Autodesk Inventor part; units mm, degrees
(part 3 of 4)
  line L1892 (-2.7113, 2.6703) -> (-2.8783, 2.4896)
  line L1893 (-2.7113, 2.6703) -> (-2.5443, 2.4896)
  line L1894 (-2.5443, 2.4896) -> (-2.7113, 2.3035)
  line L1895 (-2.8783, 2.4896) -> (-2.7113, 2.3035)
  line L1896 (-3.2281, 2.6703) -> (-3.0611, 2.4896)
  line L1897 (-3.2281, 2.6703) -> (-3.3951, 2.4896)
  line L1898 (-3.0611, 2.4896) -> (-3.2281, 2.3035)
  line L1899 (-3.3951, 2.4896) -> (-3.2281, 2.3035)
  line L1900 (-2.7113, 1.1085) -> (-2.8783, 0.9278)
  line L1901 (-2.7113, 1.1085) -> (-2.5443, 0.9278)
  line L1902 (-2.8783, 0.9278) -> (-2.7113, 0.7417)
  line L1903 (-2.7113, 0.6309) -> (-2.8783, 0.4502)
  line L1904 (-2.7113, 0.6309) -> (-2.5443, 0.4502)
  line L1905 (-2.8783, 0.4502) -> (-2.7113, 0.264)
  line L1906 (-2.5443, 0.4502) -> (-2.7113, 0.264)
  line L1907 (-2.5443, 0.9278) -> (-2.7113, 0.7417)
  line L1908 (-2.7113, 1.7094) -> (-2.8783, 1.5287)
  line L1909 (-2.5443, 1.5287) -> (-2.7113, 1.3425)
  line L1910 (-2.7113, 1.7094) -> (-2.5443, 1.5287)
  line L1911 (-2.8783, 1.5287) -> (-2.7113, 1.3425)
  line L1912 (-4.3118, 1.1085) -> (-4.4788, 0.9278)
  line L1913 (-4.4788, 0.9278) -> (-4.3118, 0.7417)
  line L1914 (-4.3118, 1.1085) -> (-4.1448, 0.9278)
  line L1915 (-4.4788, 0.4502) -> (-4.3118, 0.264)
  line L1916 (-4.1448, 0.4502) -> (-4.3118, 0.264)
  line L1917 (-4.3118, 0.6309) -> (-4.1448, 0.4502)
  line L1918 (-4.1448, 0.9278) -> (-4.3118, 0.7417)
  line L1919 (-4.3118, 0.6309) -> (-4.4788, 0.4502)
  line L1920 (-2.3773, 9.764) -> (-2.5443, 9.5833)
  line L1921 (-2.5443, 9.5833) -> (-2.3773, 9.3971)
  line L1922 (-2.3773, 9.764) -> (-2.2103, 9.5833)
  line L1923 (-2.2103, 9.5833) -> (-2.3773, 9.3971)
  line L1924 (-2.3773, 9.2863) -> (-2.5443, 9.1056)
  line L1925 (-2.5443, 9.1056) -> (-2.3773, 8.9195)
  line L1926 (-2.3773, 9.2863) -> (-2.2103, 9.1056)
  line L1927 (-2.2103, 9.1056) -> (-2.3773, 8.9195)
  line L1928 (-2.3773, 8.827) -> (-2.5443, 8.6463)
  line L1929 (-2.5443, 8.6463) -> (-2.3773, 8.4602)
  line L1930 (-2.3773, 8.827) -> (-2.2103, 8.6463)
  line L1931 (-2.2103, 8.6463) -> (-2.3773, 8.4602)
  line L1932 (-2.3773, 8.3637) -> (-2.5443, 8.183)
  line L1933 (-2.5443, 8.183) -> (-2.3773, 7.9969)
  line L1934 (-2.3773, 8.3637) -> (-2.2103, 8.183)
  line L1935 (-2.2103, 8.183) -> (-2.3773, 7.9969)
  line L1936 (-2.3773, 7.8983) -> (-2.5443, 7.7177)
  line L1937 (-2.5443, 7.7177) -> (-2.3773, 7.5315)
  line L1938 (-2.3773, 7.8983) -> (-2.2103, 7.7177)
  line L1939 (-2.2103, 7.7177) -> (-2.3773, 7.5315)
  line L1940 (-2.3773, 7.4088) -> (-2.5443, 7.2281)
  line L1941 (-2.5443, 7.2281) -> (-2.3773, 7.042)
  line L1942 (-2.3773, 7.4088) -> (-2.2103, 7.2281)
  line L1943 (-2.2103, 7.2281) -> (-2.3773, 7.042)
  line L1944 (-2.3773, 6.9434) -> (-2.5443, 6.7628)
  line L1945 (-2.5443, 6.7628) -> (-2.3773, 6.5766)
  line L1946 (-2.3773, 6.9434) -> (-2.2103, 6.7628)
  line L1947 (-2.2103, 6.7628) -> (-2.3773, 6.5766)
  line L1948 (-2.3773, 6.4539) -> (-2.5443, 6.2732)
  line L1949 (-2.5443, 6.2732) -> (-2.3773, 6.0871)
  line L1950 (-2.3773, 6.4539) -> (-2.2103, 6.2732)
  line L1951 (-2.2103, 6.2732) -> (-2.3773, 6.0871)
  line L1952 (-2.3773, 5.9825) -> (-2.5443, 5.8018)
  line L1953 (-2.5443, 5.8018) -> (-2.3773, 5.6157)
  line L1954 (-2.3773, 5.9825) -> (-2.2103, 5.8018)
  line L1955 (-2.2103, 5.8018) -> (-2.3773, 5.6157)
  line L1956 (-2.3773, 5.4909) -> (-2.5443, 5.3102)
  line L1957 (-2.5443, 5.3102) -> (-2.3773, 5.124)
  line L1958 (-2.3773, 5.4909) -> (-2.2103, 5.3102)
  line L1959 (-2.3773, 4.5539) -> (-2.5443, 4.3732)
  line L1960 (-2.3773, 4.5539) -> (-2.2103, 4.3732)
  line L1961 (-2.5443, 4.8325) -> (-2.3773, 4.6463)
  line L1962 (-2.2103, 4.8325) -> (-2.3773, 4.6463)
  line L1963 (-2.3773, 5.0132) -> (-2.2103, 4.8325)
  line L1964 (-2.2103, 5.3102) -> (-2.3773, 5.124)
  line L1965 (-2.3773, 5.0132) -> (-2.5443, 4.8325)
  line L1966 (-2.5443, 4.3732) -> (-2.3773, 4.187)
  line L1967 (-2.2103, 4.3732) -> (-2.3773, 4.187)
  line L1968 (-2.3773, 4.0906) -> (-2.5443, 3.9099)
  line L1969 (-2.3773, 4.0906) -> (-2.2103, 3.9099)
  line L1970 (-2.5443, 3.9099) -> (-2.3773, 3.7237)
  line L1971 (-2.2103, 3.9099) -> (-2.3773, 3.7237)
  line L1972 (-2.3773, 3.6252) -> (-2.5443, 3.4445)
  line L1973 (-2.3773, 3.6252) -> (-2.2103, 3.4445)
  line L1974 (-2.5443, 3.4445) -> (-2.3773, 3.2584)
  line L1975 (-2.2103, 3.4445) -> (-2.3773, 3.2584)
  line L1976 (-2.3773, 3.1357) -> (-2.5443, 2.955)
  line L1977 (-2.3773, 3.1357) -> (-2.2103, 2.955)
  line L1978 (-2.5443, 2.955) -> (-2.3773, 2.7688)
  line L1979 (-2.2103, 2.955) -> (-2.3773, 2.7688)
  line L1980 (-2.3773, 2.6703) -> (-2.2103, 2.4896)
  line L1981 (-2.3773, 2.6703) -> (-2.5443, 2.4896)
  line L1982 (-2.2103, 2.4896) -> (-2.3773, 2.3035)
  line L1983 (-2.5443, 2.4896) -> (-2.3773, 2.3035)
  line L1984 (-2.3773, 2.1808) -> (-2.5443, 2.0001)
  line L1985 (-2.3773, 2.1808) -> (-2.2103, 2.0001)
  line L1986 (-2.5443, 2.0001) -> (-2.3773, 1.8139)
  line L1987 (-2.2103, 2.0001) -> (-2.3773, 1.8139)
  line L1988 (-2.3773, 1.7094) -> (-2.5443, 1.5287)
  line L1989 (-2.3773, 1.7094) -> (-2.2103, 1.5287)
  line L1990 (-2.5443, 1.5287) -> (-2.3773, 1.3425)
  line L1991 (-2.2103, 1.5287) -> (-2.3773, 1.3425)
  line L1992 (-2.3773, 1.1085) -> (-2.5443, 0.9278)
  line L1993 (-2.5443, 0.9278) -> (-2.3773, 0.7417)
  line L1994 (-2.3773, 1.1085) -> (-2.2103, 0.9278)
  line L1995 (-2.5443, 0.4502) -> (-2.3773, 0.264)
  line L1996 (-2.2103, 0.4502) -> (-2.3773, 0.264)
  line L1997 (-2.3773, 0.6309) -> (-2.2103, 0.4502)
  line L1998 (-2.2103, 0.9278) -> (-2.3773, 0.7417)
  line L1999 (-2.3773, 0.6309) -> (-2.5443, 0.4502)
  line L2000 (-1.8605, 9.764) -> (-2.0275, 9.5833)
  line L2001 (-2.0275, 9.5833) -> (-1.8605, 9.3971)
  line L2002 (-1.8605, 9.764) -> (-1.6935, 9.5833)
  line L2003 (-1.8605, 8.827) -> (-2.0275, 8.6463)
  line L2004 (-1.8605, 8.827) -> (-1.6935, 8.6463)
  line L2005 (-1.6935, 9.1056) -> (-1.8605, 8.9195)
  line L2006 (-1.8605, 9.2863) -> (-2.0275, 9.1056)
  line L2007 (-1.8605, 9.2863) -> (-1.6935, 9.1056)
  line L2008 (-1.6935, 9.5833) -> (-1.8605, 9.3971)
  line L2009 (-2.0275, 9.1056) -> (-1.8605, 8.9195)
  line L2010 (-2.0275, 8.6463) -> (-1.8605, 8.4602)
  line L2011 (-1.6935, 8.6463) -> (-1.8605, 8.4602)
  line L2012 (-1.8605, 8.3637) -> (-2.0275, 8.183)
  line L2013 (-1.8605, 8.3637) -> (-1.6935, 8.183)
  line L2014 (-2.0275, 8.183) -> (-1.8605, 7.9969)
  line L2015 (-1.6935, 8.183) -> (-1.8605, 7.9969)
  line L2016 (-1.8605, 7.8983) -> (-2.0275, 7.7177)
  line L2017 (-2.0275, 7.7177) -> (-1.8605, 7.5315)
  line L2018 (-1.6935, 7.7177) -> (-1.8605, 7.5315)
  line L2019 (-1.8605, 7.8983) -> (-1.6935, 7.7177)
  line L2020 (-1.8605, 7.4088) -> (-1.6935, 7.2281)
  line L2021 (-1.8605, 7.4088) -> (-2.0275, 7.2281)
  line L2022 (-2.0275, 7.2281) -> (-1.8605, 7.042)
  line L2023 (-1.6935, 7.2281) -> (-1.8605, 7.042)
  line L2024 (-1.8605, 6.9434) -> (-1.6935, 6.7628)
  line L2025 (-1.6935, 6.7628) -> (-1.8605, 6.5766)
  line L2026 (-2.0275, 6.7628) -> (-1.8605, 6.5766)
  line L2027 (-1.8605, 6.9434) -> (-2.0275, 6.7628)
  line L2028 (-1.8605, 6.4539) -> (-2.0275, 6.2732)
  line L2029 (-1.8605, 6.4539) -> (-1.6935, 6.2732)
  line L2030 (-2.0275, 6.2732) -> (-1.8605, 6.0871)
  line L2031 (-1.6935, 6.2732) -> (-1.8605, 6.0871)
  line L2032 (-1.8605, 5.9825) -> (-2.0275, 5.8018)
  line L2033 (-1.8605, 5.9825) -> (-1.6935, 5.8018)
  line L2034 (-2.0275, 5.8018) -> (-1.8605, 5.6157)
  line L2035 (-1.6935, 5.8018) -> (-1.8605, 5.6157)
  line L2036 (-1.8605, 5.4909) -> (-2.0275, 5.3102)
  line L2037 (-1.8605, 5.4909) -> (-1.6935, 5.3102)
  line L2038 (-2.0275, 5.3102) -> (-1.8605, 5.124)
  line L2039 (-1.6935, 5.3102) -> (-1.8605, 5.124)
  line L2040 (-1.8605, 5.0132) -> (-2.0275, 4.8325)
  line L2041 (-1.8605, 5.0132) -> (-1.6935, 4.8325)
  line L2042 (-2.0275, 4.8325) -> (-1.8605, 4.6463)
  line L2043 (-1.6935, 4.8325) -> (-1.8605, 4.6463)
  line L2044 (-1.8605, 4.5539) -> (-1.6935, 4.3732)
  line L2045 (-1.8605, 4.5539) -> (-2.0275, 4.3732)
  line L2046 (-2.0275, 4.3732) -> (-1.8605, 4.187)
  line L2047 (-1.6935, 4.3732) -> (-1.8605, 4.187)
  line L2048 (-1.8605, 4.0906) -> (-2.0275, 3.9099)
  line L2049 (-1.8605, 4.0906) -> (-1.6935, 3.9099)
  line L2050 (-2.0275, 3.9099) -> (-1.8605, 3.7237)
  line L2051 (-1.6935, 3.9099) -> (-1.8605, 3.7237)
  line L2052 (-1.8605, 3.6252) -> (-2.0275, 3.4445)
  line L2053 (-1.8605, 3.6252) -> (-1.6935, 3.4445)
  line L2054 (-2.0275, 3.4445) -> (-1.8605, 3.2584)
  line L2055 (-1.6935, 3.4445) -> (-1.8605, 3.2584)
  line L2056 (-1.8605, 3.1357) -> (-2.0275, 2.955)
  line L2057 (-1.8605, 3.1357) -> (-1.6935, 2.955)
  line L2058 (-2.0275, 2.955) -> (-1.8605, 2.7688)
  line L2059 (-1.6935, 2.955) -> (-1.8605, 2.7688)
  line L2060 (-1.8605, 2.6703) -> (-1.6935, 2.4896)
  line L2061 (-1.8605, 2.6703) -> (-2.0275, 2.4896)
  line L2062 (-2.0275, 2.4896) -> (-1.8605, 2.3035)
  line L2063 (-1.6935, 2.4896) -> (-1.8605, 2.3035)
  line L2064 (-1.8605, 1.1085) -> (-2.0275, 0.9278)
  line L2065 (-1.8605, 1.1085) -> (-1.6935, 0.9278)
  line L2066 (-2.0275, 0.9278) -> (-1.8605, 0.7417)
  line L2067 (-1.8605, 0.6309) -> (-1.6935, 0.4502)
  line L2068 (-1.8605, 0.6309) -> (-2.0275, 0.4502)
  line L2069 (-2.0275, 0.4502) -> (-1.8605, 0.264)
  line L2070 (-1.6935, 0.4502) -> (-1.8605, 0.264)
  line L2071 (-1.6935, 0.9278) -> (-1.8605, 0.7417)
  line L2072 (-1.8605, 2.1808) -> (-1.6935, 2.0001)
  line L2073 (-1.8605, 2.1808) -> (-2.0275, 2.0001)
  line L2074 (-2.0275, 2.0001) -> (-1.8605, 1.8139)
  line L2075 (-1.6935, 2.0001) -> (-1.8605, 1.8139)
  line L2076 (-1.8605, 1.7094) -> (-1.6935, 1.5287)
  line L2077 (-1.8605, 1.7094) -> (-2.0275, 1.5287)
  line L2078 (-1.6935, 1.5287) -> (-1.8605, 1.3425)
  line L2079 (-2.0275, 1.5287) -> (-1.8605, 1.3425)
  line L2080 (-0.7767, 9.2863) -> (-0.9437, 9.1056)
  line L2081 (-0.7767, 9.2863) -> (-0.6097, 9.1056)
  line L2082 (-0.6097, 9.1056) -> (-0.7767, 8.9195)
  line L2083 (-0.9437, 9.1056) -> (-0.7767, 8.9195)
  line L2084 (-0.7767, 8.827) -> (-0.6097, 8.6463)
  line L2085 (-0.7767, 8.827) -> (-0.9437, 8.6463)
  line L2086 (-1.2936, 9.2863) -> (-1.1266, 9.1056)
  line L2087 (-1.2936, 9.2863) -> (-1.4605, 9.1056)
  line L2088 (-1.1266, 9.1056) -> (-1.2936, 8.9195)
  line L2089 (-1.4605, 9.1056) -> (-1.2936, 8.9195)
  line L2090 (-1.2936, 9.764) -> (-1.4605, 9.5833)
  line L2091 (-1.4605, 9.5833) -> (-1.2936, 9.3971)
  line L2092 (-1.1266, 9.5833) -> (-1.2936, 9.3971)
  line L2093 (-1.2936, 9.764) -> (-1.1266, 9.5833)
  line L2094 (-0.9437, 9.5833) -> (-0.7767, 9.3971)
  line L2095 (-0.6097, 9.5833) -> (-0.7767, 9.3971)
  line L2096 (-0.7767, 9.764) -> (-0.9437, 9.5833)
  line L2097 (-0.7767, 9.764) -> (-0.6097, 9.5833)
  line L2098 (-1.2936, 7.4088) -> (-1.4605, 7.2281)
  line L2099 (-1.4605, 7.2281) -> (-1.2936, 7.042)
  line L2100 (-1.2936, 6.4539) -> (-1.1266, 6.2732)
  line L2101 (-1.2936, 6.4539) -> (-1.4605, 6.2732)
  line L2102 (-1.1266, 6.2732) -> (-1.2936, 6.0871)
  line L2103 (-1.4605, 6.2732) -> (-1.2936, 6.0871)
  line L2104 (-0.7767, 5.9825) -> (-0.6097, 5.8018)
  line L2105 (-0.7767, 5.9825) -> (-0.9437, 5.8018)
  line L2106 (-0.6097, 5.8018) -> (-0.7767, 5.6157)
  line L2107 (-0.9437, 5.8018) -> (-0.7767, 5.6157)
  line L2108 (-1.2936, 5.9825) -> (-1.1266, 5.8018)
  line L2109 (-1.2936, 5.9825) -> (-1.4605, 5.8018)
  line L2110 (-1.1266, 5.8018) -> (-1.2936, 5.6157)
  line L2111 (-1.4605, 5.8018) -> (-1.2936, 5.6157)
  line L2112 (-0.9437, 4.8325) -> (-0.7767, 4.6463)
  line L2113 (-0.6097, 4.8325) -> (-0.7767, 4.6463)
  line L2114 (-1.2936, 5.0132) -> (-1.1266, 4.8325)
  line L2115 (-1.2936, 5.0132) -> (-1.4605, 4.8325)
  line L2116 (-0.7767, 4.5539) -> (-0.6097, 4.3732)
  line L2117 (-0.7767, 4.5539) -> (-0.9437, 4.3732)
  line L2118 (-1.1266, 4.8325) -> (-1.2936, 4.6463)
  line L2119 (-1.4605, 4.8325) -> (-1.2936, 4.6463)
  line L2120 (-1.2936, 4.5539) -> (-1.1266, 4.3732)
  line L2121 (-1.2936, 4.5539) -> (-1.4605, 4.3732)
  line L2122 (-1.1266, 3.4445) -> (-1.2936, 3.2584)
  line L2123 (-1.4605, 3.4445) -> (-1.2936, 3.2584)
  line L2124 (-1.2936, 3.6252) -> (-1.1266, 3.4445)
  line L2125 (-1.2936, 3.6252) -> (-1.4605, 3.4445)
  line L2126 (-1.4605, 3.9099) -> (-1.2936, 3.7237)
  line L2127 (-1.2936, 4.0906) -> (-1.1266, 3.9099)
  line L2128 (-1.2936, 4.0906) -> (-1.4605, 3.9099)
  line L2129 (-1.1266, 3.9099) -> (-1.2936, 3.7237)
  line L2130 (-1.2936, 8.827) -> (-1.4605, 8.6463)
  line L2131 (-1.4605, 8.6463) -> (-1.2936, 8.4602)
  line L2132 (-1.2936, 8.827) -> (-1.1266, 8.6463)
  line L2133 (-1.1266, 8.6463) -> (-1.2936, 8.4602)
  line L2134 (-1.2936, 8.3637) -> (-1.4605, 8.183)
  line L2135 (-1.4605, 8.183) -> (-1.2936, 7.9969)
  line L2136 (-1.2936, 8.3637) -> (-1.1266, 8.183)
  line L2137 (-0.6097, 8.6463) -> (-0.7767, 8.4602)
  line L2138 (-0.9437, 8.6463) -> (-0.7767, 8.4602)
  line L2139 (-0.7767, 8.3637) -> (-0.6097, 8.183)
  line L2140 (-0.6097, 8.183) -> (-0.7767, 7.9969)
  line L2141 (-0.9437, 8.183) -> (-0.7767, 7.9969)
  line L2142 (-1.1266, 8.183) -> (-1.2936, 7.9969)
  line L2143 (-0.7767, 8.3637) -> (-0.9437, 8.183)
  line L2144 (-1.2936, 7.8983) -> (-1.4605, 7.7177)
  line L2145 (-1.4605, 7.7177) -> (-1.2936, 7.5315)
  line L2146 (-1.2936, 7.4088) -> (-1.1266, 7.2281)
  line L2147 (-1.1266, 7.2281) -> (-1.2936, 7.042)
  line L2148 (-1.1266, 7.7177) -> (-1.2936, 7.5315)
  line L2149 (-1.2936, 7.8983) -> (-1.1266, 7.7177)
  line L2150 (-0.7767, 6.9434) -> (-0.9437, 6.7628)
  line L2151 (-0.7767, 6.9434) -> (-0.6097, 6.7628)
  line L2152 (-0.7767, 7.4088) -> (-0.9437, 7.2281)
  line L2153 (-0.6097, 7.2281) -> (-0.7767, 7.042)
  line L2154 (-0.9437, 7.7177) -> (-0.7767, 7.5315)
  line L2155 (-0.7767, 7.8983) -> (-0.9437, 7.7177)
  line L2156 (-0.7767, 7.8983) -> (-0.6097, 7.7177)
  line L2157 (-0.6097, 7.7177) -> (-0.7767, 7.5315)
  line L2158 (-0.7767, 7.4088) -> (-0.6097, 7.2281)
  line L2159 (-0.9437, 7.2281) -> (-0.7767, 7.042)
  line L2160 (-1.2936, 6.9434) -> (-1.4605, 6.7628)
  line L2161 (-1.4605, 6.7628) -> (-1.2936, 6.5766)
  line L2162 (-1.2936, 6.9434) -> (-1.1266, 6.7628)
  line L2163 (-1.1266, 6.7628) -> (-1.2936, 6.5766)
  line L2164 (-0.9437, 6.2732) -> (-0.7767, 6.0871)
  line L2165 (-0.6097, 6.2732) -> (-0.7767, 6.0871)
  line L2166 (-0.7767, 6.4539) -> (-0.9437, 6.2732)
  line L2167 (-0.7767, 6.4539) -> (-0.6097, 6.2732)
  line L2168 (-0.9437, 6.7628) -> (-0.7767, 6.5766)
  line L2169 (-0.6097, 6.7628) -> (-0.7767, 6.5766)
  line L2170 (-1.2936, 5.4909) -> (-1.4605, 5.3102)
  line L2171 (-1.4605, 5.3102) -> (-1.2936, 5.124)
  line L2172 (-1.2936, 5.4909) -> (-1.1266, 5.3102)
  line L2173 (-0.7767, 5.0132) -> (-0.9437, 4.8325)
  line L2174 (-1.1266, 5.3102) -> (-1.2936, 5.124)
  line L2175 (-0.9437, 5.3102) -> (-0.7767, 5.124)
  line L2176 (-0.6097, 5.3102) -> (-0.7767, 5.124)
  line L2177 (-0.7767, 5.4909) -> (-0.9437, 5.3102)
  line L2178 (-0.7767, 5.4909) -> (-0.6097, 5.3102)
  line L2179 (-0.7767, 5.0132) -> (-0.6097, 4.8325)
  line L2180 (-1.4605, 4.3732) -> (-1.2936, 4.187)
  line L2181 (-1.1266, 4.3732) -> (-1.2936, 4.187)
  line L2182 (-0.9437, 4.3732) -> (-0.7767, 4.187)
  line L2183 (-0.6097, 4.3732) -> (-0.7767, 4.187)
  line L2184 (-0.7767, 4.0906) -> (-0.9437, 3.9099)
  line L2185 (-0.7767, 4.0906) -> (-0.6097, 3.9099)
  line L2186 (-0.6097, 3.9099) -> (-0.7767, 3.7237)
  line L2187 (-0.7767, 3.6252) -> (-0.9437, 3.4445)
  line L2188 (-0.7767, 3.6252) -> (-0.6097, 3.4445)
  line L2189 (-0.9437, 3.4445) -> (-0.7767, 3.2584)
  line L2190 (-0.6097, 3.4445) -> (-0.7767, 3.2584)
  line L2191 (-0.9437, 3.9099) -> (-0.7767, 3.7237)
  line L2192 (-1.2936, 3.1357) -> (-1.4605, 2.955)
  line L2193 (-1.2936, 3.1357) -> (-1.1266, 2.955)
  line L2194 (-1.4605, 2.955) -> (-1.2936, 2.7688)
  line L2195 (-1.1266, 2.955) -> (-1.2936, 2.7688)
  line L2196 (-1.2936, 2.6703) -> (-1.1266, 2.4896)
  line L2197 (-1.2936, 2.6703) -> (-1.4605, 2.4896)
  line L2198 (-1.1266, 2.4896) -> (-1.2936, 2.3035)
  line L2199 (-1.4605, 2.4896) -> (-1.2936, 2.3035)
  line L2200 (-0.7767, 3.1357) -> (-0.9437, 2.955)
  line L2201 (-0.7767, 3.1357) -> (-0.6097, 2.955)
  line L2202 (-0.9437, 2.955) -> (-0.7767, 2.7688)
  line L2203 (-0.6097, 2.955) -> (-0.7767, 2.7688)
  line L2204 (-0.7767, 2.6703) -> (-0.6097, 2.4896)
  line L2205 (-0.7767, 2.6703) -> (-0.9437, 2.4896)
  line L2206 (-0.6097, 2.4896) -> (-0.7767, 2.3035)
  line L2207 (-0.9437, 2.4896) -> (-0.7767, 2.3035)
  line L2208 (-1.2936, 2.1808) -> (-1.4605, 2.0001)
  line L2209 (-1.2936, 2.1808) -> (-1.1266, 2.0001)
  line L2210 (-1.4605, 2.0001) -> (-1.2936, 1.8139)
  line L2211 (-1.1266, 2.0001) -> (-1.2936, 1.8139)
  line L2212 (-1.2936, 1.7094) -> (-1.4605, 1.5287)
  line L2213 (-1.2936, 1.7094) -> (-1.1266, 1.5287)
  line L2214 (-1.4605, 1.5287) -> (-1.2936, 1.3425)
  line L2215 (-1.1266, 1.5287) -> (-1.2936, 1.3425)
  line L2216 (-0.7767, 2.1808) -> (-0.6097, 2.0001)
  line L2217 (-0.7767, 2.1808) -> (-0.9437, 2.0001)
  line L2218 (-0.9437, 2.0001) -> (-0.7767, 1.8139)
  line L2219 (-0.6097, 2.0001) -> (-0.7767, 1.8139)
  line L2220 (-0.7767, 1.7094) -> (-0.6097, 1.5287)
  line L2221 (-0.7767, 1.7094) -> (-0.9437, 1.5287)
  line L2222 (-0.6097, 1.5287) -> (-0.7767, 1.3425)
  line L2223 (-0.9437, 1.5287) -> (-0.7767, 1.3425)
  line L2224 (-1.2936, 1.1085) -> (-1.4605, 0.9278)
  line L2225 (-1.4605, 0.9278) -> (-1.2936, 0.7417)
  line L2226 (-1.2936, 1.1085) -> (-1.1266, 0.9278)
  line L2227 (-1.4605, 0.4502) -> (-1.2936, 0.264)
  line L2228 (-1.1266, 0.4502) -> (-1.2936, 0.264)
  line L2229 (-1.2936, 0.6309) -> (-1.1266, 0.4502)
  line L2230 (-1.1266, 0.9278) -> (-1.2936, 0.7417)
  line L2231 (-1.2936, 0.6309) -> (-1.4605, 0.4502)
  line L2232 (-0.7767, 1.1085) -> (-0.9437, 0.9278)
  line L2233 (-0.7767, 1.1085) -> (-0.6097, 0.9278)
  line L2234 (-0.9437, 0.9278) -> (-0.7767, 0.7417)
  line L2235 (-0.6097, 0.9278) -> (-0.7767, 0.7417)
  line L2236 (-0.7767, 0.6309) -> (-0.6097, 0.4502)
  line L2237 (-0.7767, 0.6309) -> (-0.9437, 0.4502)
  line L2238 (-0.9437, 0.4502) -> (-0.7767, 0.264)
  line L2239 (-0.6097, 0.4502) -> (-0.7767, 0.264)
  line L2240 (-0.124, 8.827) -> (-0.291, 8.6463)
  line L2241 (-0.124, 8.827) -> (0.043, 8.6463)
  line L2242 (-0.291, 8.6463) -> (-0.124, 8.4602)
  line L2243 (0.2259, 8.6463) -> (0.3929, 8.4602)
  line L2244 (0.5599, 8.6463) -> (0.3929, 8.4602)
  line L2245 (0.3929, 8.3637) -> (0.5599, 8.183)
  line L2246 (0.3929, 8.3637) -> (0.2259, 8.183)
  line L2247 (0.043, 8.6463) -> (-0.124, 8.4602)
  line L2248 (-0.291, 9.1056) -> (-0.124, 8.9195)
  line L2249 (0.043, 9.1056) -> (-0.124, 8.9195)
  line L2250 (-0.124, 9.2863) -> (-0.291, 9.1056)
  line L2251 (-0.124, 9.2863) -> (0.043, 9.1056)
  line L2252 (-0.291, 9.5833) -> (-0.124, 9.3971)
  line L2253 (-0.124, 9.764) -> (0.043, 9.5833)
  line L2254 (-0.124, 9.764) -> (-0.291, 9.5833)
  line L2255 (0.043, 9.5833) -> (-0.124, 9.3971)
  line L2256 (0.5599, 7.7177) -> (0.3929, 7.5315)
  line L2257 (-0.291, 5.8018) -> (-0.124, 5.6157)
  line L2258 (0.043, 5.8018) -> (-0.124, 5.6157)
  line L2259 (-0.124, 5.4909) -> (-0.291, 5.3102)
  line L2260 (-0.124, 5.4909) -> (0.043, 5.3102)
  line L2261 (0.3929, 5.4909) -> (0.2259, 5.3102)
  line L2262 (0.043, 5.3102) -> (-0.124, 5.124)
  line L2263 (0.3929, 5.4909) -> (0.5599, 5.3102)
  line L2264 (0.2259, 5.3102) -> (0.3929, 5.124)
  line L2265 (0.5599, 5.3102) -> (0.3929, 5.124)
  line L2266 (-0.291, 5.3102) -> (-0.124, 5.124)
  line L2267 (-0.124, 4.5539) -> (-0.291, 4.3732)
  line L2268 (-0.124, 4.5539) -> (0.043, 4.3732)
  line L2269 (-0.291, 4.8325) -> (-0.124, 4.6463)
  line L2270 (-0.124, 5.0132) -> (0.043, 4.8325)
  line L2271 (0.3929, 5.0132) -> (0.2259, 4.8325)
  line L2272 (0.3929, 5.0132) -> (0.5599, 4.8325)
  line L2273 (-0.124, 5.0132) -> (-0.291, 4.8325)
  line L2274 (0.043, 4.8325) -> (-0.124, 4.6463)
  line L2275 (0.5599, 4.8325) -> (0.3929, 4.6463)
  line L2276 (0.2259, 4.8325) -> (0.3929, 4.6463)
  line L2277 (-0.291, 4.3732) -> (-0.124, 4.187)
  line L2278 (0.043, 4.3732) -> (-0.124, 4.187)
  line L2279 (0.3929, 4.5539) -> (0.2259, 4.3732)
  line L2280 (0.3929, 4.5539) -> (0.5599, 4.3732)
  line L2281 (0.2259, 4.3732) -> (0.3929, 4.187)
  line L2282 (0.5599, 4.3732) -> (0.3929, 4.187)
  line L2283 (0.3929, 2.6703) -> (0.5599, 2.4896)
  line L2284 (0.3929, 2.6703) -> (0.2259, 2.4896)
  line L2285 (0.2259, 2.4896) -> (0.3929, 2.3035)
  line L2286 (0.5599, 2.4896) -> (0.3929, 2.3035)
  line L2287 (0.3929, 2.1808) -> (0.2259, 2.0001)
  line L2288 (0.3929, 2.1808) -> (0.5599, 2.0001)
  line L2289 (0.2259, 2.0001) -> (0.3929, 1.8139)
  line L2290 (0.5599, 2.0001) -> (0.3929, 1.8139)
  line L2291 (0.7928, 2.0001) -> (0.9598, 1.8139)
  line L2292 (0.9598, 1.7094) -> (0.7928, 1.5287)
  line L2293 (0.7928, 1.5287) -> (0.9598, 1.3425)
  line L2294 (1.1268, 1.5287) -> (0.9598, 1.3425)
  line L2295 (0.9598, 1.7094) -> (1.1268, 1.5287)
  line L2296 (0.9598, 2.1808) -> (0.7928, 2.0001)
  line L2297 (1.1268, 2.0001) -> (0.9598, 1.8139)
  line L2298 (0.9598, 2.1808) -> (1.1268, 2.0001)
  line L2299 (0.3929, 0.6309) -> (0.2259, 0.4502)
  line L2300 (0.2259, 0.4502) -> (0.3929, 0.264)
  line L2301 (0.2259, 0.9278) -> (0.3929, 0.7417)
  line L2302 (0.3929, 1.1085) -> (0.2259, 0.9278)
  line L2303 (0.3929, 0.6309) -> (0.5599, 0.4502)
  line L2304 (0.5599, 0.9278) -> (0.3929, 0.7417)
  line L2305 (0.3929, 1.1085) -> (0.5599, 0.9278)
  line L2306 (0.9598, 0.6309) -> (0.7928, 0.4502)
  line L2307 (0.7928, 0.4502) -> (0.9598, 0.264)
  line L2308 (0.7928, 0.9278) -> (0.9598, 0.7417)
  line L2309 (0.9598, 1.1085) -> (0.7928, 0.9278)
  line L2310 (0.9598, 1.1085) -> (1.1268, 0.9278)
  line L2311 (1.1268, 0.9278) -> (0.9598, 0.7417)
  line L2312 (0.9598, 0.6309) -> (1.1268, 0.4502)
  line L2313 (1.1268, 0.4502) -> (0.9598, 0.264)
  line L2314 (0.5599, 0.4502) -> (0.3929, 0.264)
  line L2315 (0.5599, 8.183) -> (0.3929, 7.9969)
  line L2316 (0.2259, 8.183) -> (0.3929, 7.9969)
  line L2317 (-0.124, 8.3637) -> (0.043, 8.183)
  line L2318 (-0.124, 8.3637) -> (-0.291, 8.183)
  line L2319 (0.3929, 7.8983) -> (0.5599, 7.7177)
  line L2320 (0.043, 8.183) -> (-0.124, 7.9969)
  line L2321 (-0.291, 8.183) -> (-0.124, 7.9969)
  line L2322 (0.3929, 7.8983) -> (0.2259, 7.7177)
  line L2323 (-0.124, 7.8983) -> (0.043, 7.7177)
  line L2324 (0.2259, 7.7177) -> (0.3929, 7.5315)
  line L2325 (-0.124, 7.8983) -> (-0.291, 7.7177)
  line L2326 (-0.291, 7.7177) -> (-0.124, 7.5315)
  line L2327 (0.043, 7.7177) -> (-0.124, 7.5315)
  line L2328 (1.1268, 6.7628) -> (0.9598, 6.5766)
  line L2329 (0.9598, 6.9434) -> (1.1268, 6.7628)
  line L2330 (0.9598, 6.4539) -> (0.7928, 6.2732)
  line L2331 (0.7928, 6.2732) -> (0.9598, 6.0871)
  line L2332 (0.9598, 6.4539) -> (1.1268, 6.2732)
  line L2333 (1.3096, 6.7628) -> (1.4766, 6.5766)
  line L2334 (1.4766, 6.9434) -> (1.3096, 6.7628)
  line L2335 (1.4766, 6.9434) -> (1.6436, 6.7628)
  line L2336 (1.6436, 6.7628) -> (1.4766, 6.5766)
  line L2337 (1.4766, 6.4539) -> (1.3096, 6.2732)
  line L2338 (1.4766, 6.4539) -> (1.6436, 6.2732)
  line L2339 (1.1268, 6.2732) -> (0.9598, 6.0871)
  line L2340 (-0.124, 7.4088) -> (-0.291, 7.2281)
  line L2341 (-0.291, 7.2281) -> (-0.124, 7.042)
  line L2342 (-0.124, 7.4088) -> (0.043, 7.2281)
  line L2343 (0.043, 7.2281) -> (-0.124, 7.042)
  line L2344 (0.3929, 7.4088) -> (0.5599, 7.2281)
  line L2345 (0.3929, 7.4088) -> (0.2259, 7.2281)
  line L2346 (0.2259, 7.2281) -> (0.3929, 7.042)
  line L2347 (0.5599, 7.2281) -> (0.3929, 7.042)
  line L2348 (0.7928, 6.7628) -> (0.9598, 6.5766)
  line L2349 (0.5599, 6.7628) -> (0.3929, 6.5766)
  line L2350 (0.3929, 6.9434) -> (0.5599, 6.7628)
  line L2351 (0.2259, 6.7628) -> (0.3929, 6.5766)
  line L2352 (0.3929, 6.9434) -> (0.2259, 6.7628)
  line L2353 (0.9598, 6.9434) -> (0.7928, 6.7628)
  line L2354 (1.4766, 5.9825) -> (1.3096, 5.8018)
  line L2355 (1.3096, 5.8018) -> (1.4766, 5.6157)
  line L2356 (1.6436, 5.8018) -> (1.4766, 5.6157)
  line L2357 (1.4766, 5.9825) -> (1.6436, 5.8018)
  line L2358 (-0.124, 6.9434) -> (-0.291, 6.7628)
  line L2359 (-0.291, 6.7628) -> (-0.124, 6.5766)
  line L2360 (-0.124, 6.9434) -> (0.043, 6.7628)
  line L2361 (0.043, 6.7628) -> (-0.124, 6.5766)
  line L2362 (-0.124, 5.9825) -> (-0.291, 5.8018)
  line L2363 (-0.124, 5.9825) -> (0.043, 5.8018)
  line L2364 (0.043, 6.2732) -> (-0.124, 6.0871)
  line L2365 (-0.124, 6.4539) -> (-0.291, 6.2732)
  line L2366 (-0.124, 6.4539) -> (0.043, 6.2732)
  line L2367 (-0.291, 6.2732) -> (-0.124, 6.0871)
  line L2368 (-0.124, 4.0906) -> (-0.291, 3.9099)
  line L2369 (-0.124, 4.0906) -> (0.043, 3.9099)
  line L2370 (-0.291, 3.9099) -> (-0.124, 3.7237)
  line L2371 (0.043, 3.9099) -> (-0.124, 3.7237)
  line L2372 (0.3929, 4.0906) -> (0.2259, 3.9099)
  line L2373 (0.3929, 4.0906) -> (0.5599, 3.9099)
  line L2374 (0.2259, 3.9099) -> (0.3929, 3.7237)
  line L2375 (0.5599, 3.9099) -> (0.3929, 3.7237)
  line L2376 (0.3929, 3.6252) -> (0.2259, 3.4445)
  line L2377 (0.3929, 3.6252) -> (0.5599, 3.4445)
  line L2378 (0.2259, 3.4445) -> (0.3929, 3.2584)
  line L2379 (0.5599, 3.4445) -> (0.3929, 3.2584)
  line L2380 (0.7928, 3.4445) -> (0.9598, 3.2584)
  line L2381 (0.9598, 3.6252) -> (0.7928, 3.4445)
  line L2382 (-0.124, 2.1808) -> (-0.291, 2.0001)
  line L2383 (-0.124, 2.1808) -> (0.043, 2.0001)
  line L2384 (-0.291, 2.0001) -> (-0.124, 1.8139)
  line L2385 (0.3929, 1.7094) -> (0.5599, 1.5287)
  line L2386 (0.5599, 1.5287) -> (0.3929, 1.3425)
  line L2387 (0.3929, 1.7094) -> (0.2259, 1.5287)
  line L2388 (0.2259, 1.5287) -> (0.3929, 1.3425)
  line L2389 (-0.124, 1.7094) -> (0.043, 1.5287)
  line L2390 (0.043, 1.5287) -> (-0.124, 1.3425)
  line L2391 (-0.124, 1.7094) -> (-0.291, 1.5287)
  line L2392 (-0.291, 1.5287) -> (-0.124, 1.3425)
  line L2393 (0.043, 2.0001) -> (-0.124, 1.8139)
  line L2394 (-0.124, 3.6252) -> (-0.291, 3.4445)
  line L2395 (-0.124, 3.6252) -> (0.043, 3.4445)
  line L2396 (-0.291, 3.4445) -> (-0.124, 3.2584)
  line L2397 (0.043, 3.4445) -> (-0.124, 3.2584)
  line L2398 (-0.124, 3.1357) -> (-0.291, 2.955)
  line L2399 (-0.124, 3.1357) -> (0.043, 2.955)
  line L2400 (-0.291, 2.955) -> (-0.124, 2.7688)
  line L2401 (0.043, 2.4896) -> (-0.124, 2.3035)
  line L2402 (-0.291, 2.4896) -> (-0.124, 2.3035)
  line L2403 (-0.124, 2.6703) -> (0.043, 2.4896)
  line L2404 (-0.124, 2.6703) -> (-0.291, 2.4896)
  line L2405 (0.2259, 2.955) -> (0.3929, 2.7688)
  line L2406 (0.5599, 2.955) -> (0.3929, 2.7688)
  line L2407 (0.3929, 3.1357) -> (0.5599, 2.955)
  line L2408 (0.3929, 3.1357) -> (0.2259, 2.955)
  line L2409 (0.043, 2.955) -> (-0.124, 2.7688)
  line L2410 (0.3929, 9.764) -> (0.2259, 9.5833)
  line L2411 (0.2259, 9.5833) -> (0.3929, 9.3971)
  line L2412 (0.3929, 9.764) -> (0.5599, 9.5833)
  line L2413 (0.3929, 8.827) -> (0.2259, 8.6463)
  line L2414 (0.3929, 8.827) -> (0.5599, 8.6463)
  line L2415 (0.5599, 9.1056) -> (0.3929, 8.9195)
  line L2416 (0.3929, 9.2863) -> (0.2259, 9.1056)
  line L2417 (0.3929, 9.2863) -> (0.5599, 9.1056)
  line L2418 (0.5599, 9.5833) -> (0.3929, 9.3971)
  line L2419 (0.2259, 9.1056) -> (0.3929, 8.9195)
  line L2420 (1.1268, 9.1056) -> (0.9598, 8.9195)
  line L2421 (0.7928, 9.1056) -> (0.9598, 8.9195)
  line L2422 (1.4766, 9.2863) -> (1.3096, 9.1056)
  line L2423 (1.4766, 9.2863) -> (1.6436, 9.1056)
  line L2424 (1.6436, 9.1056) -> (1.4766, 8.9195)
  line L2425 (1.3096, 9.1056) -> (1.4766, 8.9195)
  line L2426 (0.9598, 9.2863) -> (1.1268, 9.1056)
  line L2427 (0.9598, 9.2863) -> (0.7928, 9.1056)
  line L2428 (0.9598, 9.764) -> (0.7928, 9.5833)
  line L2429 (0.7928, 9.5833) -> (0.9598, 9.3971)
  line L2430 (1.1268, 9.5833) -> (0.9598, 9.3971)
  line L2431 (0.9598, 9.764) -> (1.1268, 9.5833)
  line L2432 (1.3096, 9.5833) -> (1.4766, 9.3971)
  line L2433 (1.6436, 9.5833) -> (1.4766, 9.3971)
  line L2434 (1.4766, 9.764) -> (1.3096, 9.5833)
  line L2435 (1.4766, 9.764) -> (1.6436, 9.5833)
  line L2436 (1.4766, 5.4909) -> (1.3096, 5.3102)
  line L2437 (1.4766, 5.4909) -> (1.6436, 5.3102)
  line L2438 (1.3096, 5.3102) -> (1.4766, 5.124)
  line L2439 (1.6436, 5.3102) -> (1.4766, 5.124)
  line L2440 (0.9598, 5.0132) -> (1.1268, 4.8325)
  line L2441 (0.9598, 5.0132) -> (0.7928, 4.8325)
  line L2442 (0.7928, 4.8325) -> (0.9598, 4.6463)
  line L2443 (1.1268, 4.8325) -> (0.9598, 4.6463)
  line L2444 (1.4766, 5.0132) -> (1.3096, 4.8325)
  line L2445 (1.4766, 5.0132) -> (1.6436, 4.8325)
  line L2446 (1.3096, 4.8325) -> (1.4766, 4.6463)
  line L2447 (1.6436, 4.8325) -> (1.4766, 4.6463)
  line L2448 (1.4766, 4.5539) -> (1.6436, 4.3732)
  line L2449 (1.4766, 4.5539) -> (1.3096, 4.3732)
  line L2450 (0.9598, 4.5539) -> (1.1268, 4.3732)
  line L2451 (0.9598, 4.5539) -> (0.7928, 4.3732)
  line L2452 (1.6436, 4.3732) -> (1.4766, 4.187)
  line L2453 (0.7928, 4.3732) -> (0.9598, 4.187)
  line L2454 (1.1268, 4.3732) -> (0.9598, 4.187)
  line L2455 (1.3096, 4.3732) -> (1.4766, 4.187)
  line L2456 (1.4766, 4.0906) -> (1.6436, 3.9099)
  line L2457 (1.4766, 4.0906) -> (1.3096, 3.9099)
  line L2458 (0.9598, 4.0906) -> (1.1268, 3.9099)
  line L2459 (0.9598, 4.0906) -> (0.7928, 3.9099)
  line L2460 (0.9598, 8.827) -> (1.1268, 8.6463)
  line L2461 (0.9598, 8.827) -> (0.7928, 8.6463)
  line L2462 (1.1268, 8.6463) -> (0.9598, 8.4602)
  line L2463 (0.7928, 8.6463) -> (0.9598, 8.4602)
  line L2464 (1.4766, 8.827) -> (1.3096, 8.6463)
  line L2465 (1.4766, 8.827) -> (1.6436, 8.6463)
  line L2466 (1.3096, 8.6463) -> (1.4766, 8.4602)
  line L2467 (1.6436, 8.6463) -> (1.4766, 8.4602)
  line L2468 (0.9598, 8.3637) -> (1.1268, 8.183)
  line L2469 (0.9598, 8.3637) -> (0.7928, 8.183)
  line L2470 (0.7928, 8.183) -> (0.9598, 7.9969)
  line L2471 (1.1268, 8.183) -> (0.9598, 7.9969)
  line L2472 (1.4766, 8.3637) -> (1.3096, 8.183)
  line L2473 (1.4766, 8.3637) -> (1.6436, 8.183)
  line L2474 (1.3096, 8.183) -> (1.4766, 7.9969)
  line L2475 (1.6436, 8.183) -> (1.4766, 7.9969)
  line L2476 (0.9598, 7.8983) -> (0.7928, 7.7177)
  line L2477 (0.7928, 7.7177) -> (0.9598, 7.5315)
  line L2478 (0.9598, 7.8983) -> (1.1268, 7.7177)
  line L2479 (1.1268, 7.7177) -> (0.9598, 7.5315)
  line L2480 (1.4766, 7.8983) -> (1.3096, 7.7177)
  line L2481 (1.3096, 7.7177) -> (1.4766, 7.5315)
  line L2482 (1.4766, 7.8983) -> (1.6436, 7.7177)
  line L2483 (1.6436, 7.7177) -> (1.4766, 7.5315)
  line L2484 (0.9598, 7.4088) -> (0.7928, 7.2281)
  line L2485 (0.7928, 7.2281) -> (0.9598, 7.042)
  line L2486 (1.4766, 7.4088) -> (1.3096, 7.2281)
  line L2487 (1.4766, 7.4088) -> (1.6436, 7.2281)
  line L2488 (0.9598, 7.4088) -> (1.1268, 7.2281)
  line L2489 (1.6436, 7.2281) -> (1.4766, 7.042)
  line L2490 (1.3096, 7.2281) -> (1.4766, 7.042)
  line L2491 (1.1268, 7.2281) -> (0.9598, 7.042)
  line L2492 (1.3096, 6.2732) -> (1.4766, 6.0871)
  line L2493 (1.6436, 6.2732) -> (1.4766, 6.0871)
  line L2494 (0.7928, 3.9099) -> (0.9598, 3.7237)
  line L2495 (1.1268, 3.4445) -> (0.9598, 3.2584)
  line L2496 (0.9598, 3.6252) -> (1.1268, 3.4445)
  line L2497 (1.1268, 3.9099) -> (0.9598, 3.7237)
  line L2498 (1.3096, 3.4445) -> (1.4766, 3.2584)
  line L2499 (1.4766, 3.6252) -> (1.3096, 3.4445)
  line L2500 (1.4766, 3.1357) -> (1.3096, 2.955)
  line L2501 (1.3096, 3.9099) -> (1.4766, 3.7237)
  line L2502 (1.6436, 3.9099) -> (1.4766, 3.7237)
  line L2503 (1.4766, 3.6252) -> (1.6436, 3.4445)
  line L2504 (1.4766, 3.1357) -> (1.6436, 2.955)
  line L2505 (1.6436, 3.4445) -> (1.4766, 3.2584)
  line L2506 (0.3929, 6.4539) -> (0.2259, 6.2732)
  line L2507 (0.3929, 6.4539) -> (0.5599, 6.2732)
  line L2508 (0.2259, 6.2732) -> (0.3929, 6.0871)
  line L2509 (0.9598, 5.9825) -> (1.1268, 5.8018)
  line L2510 (1.1268, 5.8018) -> (0.9598, 5.6157)
  line L2511 (0.9598, 5.9825) -> (0.7928, 5.8018)
  line L2512 (0.7928, 5.8018) -> (0.9598, 5.6157)
  line L2513 (0.9598, 5.4909) -> (1.1268, 5.3102)
  line L2514 (1.1268, 5.3102) -> (0.9598, 5.124)
  line L2515 (0.7928, 5.3102) -> (0.9598, 5.124)
  line L2516 (0.9598, 5.4909) -> (0.7928, 5.3102)
  line L2517 (0.5599, 6.2732) -> (0.3929, 6.0871)
  line L2518 (0.3929, 5.9825) -> (0.5599, 5.8018)
  line L2519 (0.5599, 5.8018) -> (0.3929, 5.6157)
  line L2520 (0.3929, 5.9825) -> (0.2259, 5.8018)
  line L2521 (0.2259, 5.8018) -> (0.3929, 5.6157)
  line L2522 (1.4766, 2.1808) -> (1.6436, 2.0001)
  line L2523 (1.6436, 2.0001) -> (1.4766, 1.8139)
  line L2524 (1.3096, 2.0001) -> (1.4766, 1.8139)
  line L2525 (1.4766, 2.1808) -> (1.3096, 2.0001)
  line L2526 (0.9598, 3.1357) -> (1.1268, 2.955)
  line L2527 (0.9598, 3.1357) -> (0.7928, 2.955)
  line L2528 (1.3096, 2.955) -> (1.4766, 2.7688)
  line L2529 (1.6436, 2.955) -> (1.4766, 2.7688)
  line L2530 (1.1268, 2.955) -> (0.9598, 2.7688)
  line L2531 (0.7928, 2.955) -> (0.9598, 2.7688)
  line L2532 (1.4766, 2.6703) -> (1.3096, 2.4896)
  line L2533 (1.4766, 2.6703) -> (1.6436, 2.4896)
  line L2534 (1.6436, 2.4896) -> (1.4766, 2.3035)
  line L2535 (1.3096, 2.4896) -> (1.4766, 2.3035)
  line L2536 (0.9598, 2.6703) -> (1.1268, 2.4896)
  line L2537 (0.9598, 2.6703) -> (0.7928, 2.4896)
  line L2538 (1.1268, 2.4896) -> (0.9598, 2.3035)
  line L2539 (0.7928, 2.4896) -> (0.9598, 2.3035)
  line L2540 (1.4766, 1.1085) -> (1.3096, 0.9278)
  line L2541 (1.4766, 1.1085) -> (1.6436, 0.9278)
  line L2542 (1.3096, 0.9278) -> (1.4766, 0.7417)
  line L2543 (1.4766, 0.6309) -> (1.3096, 0.4502)
  line L2544 (1.4766, 0.6309) -> (1.6436, 0.4502)
  line L2545 (1.3096, 0.4502) -> (1.4766, 0.264)
  line L2546 (1.6436, 0.4502) -> (1.4766, 0.264)
  line L2547 (1.6436, 0.9278) -> (1.4766, 0.7417)
  line L2548 (1.4766, 1.7094) -> (1.3096, 1.5287)
  line L2549 (1.6436, 1.5287) -> (1.4766, 1.3425)
  line L2550 (1.4766, 1.7094) -> (1.6436, 1.5287)
  line L2551 (1.3096, 1.5287) -> (1.4766, 1.3425)
  line L2552 (-0.124, 1.1085) -> (-0.291, 0.9278)
  line L2553 (-0.291, 0.9278) -> (-0.124, 0.7417)
  line L2554 (-0.124, 1.1085) -> (0.043, 0.9278)
  line L2555 (-0.291, 0.4502) -> (-0.124, 0.264)
  line L2556 (0.043, 0.4502) -> (-0.124, 0.264)
  line L2557 (-0.124, 0.6309) -> (0.043, 0.4502)
  line L2558 (0.043, 0.9278) -> (-0.124, 0.7417)
  line L2559 (-0.124, 0.6309) -> (-0.291, 0.4502)
  line L2560 (1.8106, 9.764) -> (1.6436, 9.5833)
  line L2561 (1.6436, 9.5833) -> (1.8106, 9.3971)
  line L2562 (1.8106, 9.764) -> (1.9776, 9.5833)
  line L2563 (1.9776, 9.5833) -> (1.8106, 9.3971)
  line L2564 (1.8106, 9.2863) -> (1.6436, 9.1056)
  line L2565 (1.6436, 9.1056) -> (1.8106, 8.9195)
  line L2566 (1.8106, 9.2863) -> (1.9776, 9.1056)
  line L2567 (1.9776, 9.1056) -> (1.8106, 8.9195)
  line L2568 (1.8106, 8.827) -> (1.6436, 8.6463)
  line L2569 (1.6436, 8.6463) -> (1.8106, 8.4602)
  line L2570 (1.8106, 8.827) -> (1.9776, 8.6463)
  line L2571 (1.9776, 8.6463) -> (1.8106, 8.4602)
  line L2572 (1.8106, 8.3637) -> (1.6436, 8.183)
  line L2573 (1.6436, 8.183) -> (1.8106, 7.9969)
  line L2574 (1.8106, 8.3637) -> (1.9776, 8.183)
  line L2575 (1.9776, 8.183) -> (1.8106, 7.9969)
  line L2576 (1.8106, 7.8983) -> (1.6436, 7.7177)
  line L2577 (1.6436, 7.7177) -> (1.8106, 7.5315)
  line L2578 (1.8106, 7.8983) -> (1.9776, 7.7177)
  line L2579 (1.9776, 7.7177) -> (1.8106, 7.5315)
  line L2580 (1.8106, 7.4088) -> (1.6436, 7.2281)
  line L2581 (1.6436, 7.2281) -> (1.8106, 7.042)
  line L2582 (1.8106, 7.4088) -> (1.9776, 7.2281)
  line L2583 (1.9776, 7.2281) -> (1.8106, 7.042)
  line L2584 (1.8106, 6.9434) -> (1.6436, 6.7628)
  line L2585 (1.6436, 6.7628) -> (1.8106, 6.5766)
  line L2586 (1.8106, 6.9434) -> (1.9776, 6.7628)
  line L2587 (1.9776, 6.7628) -> (1.8106, 6.5766)
  line L2588 (1.8106, 6.4539) -> (1.6436, 6.2732)
  line L2589 (1.6436, 6.2732) -> (1.8106, 6.0871)
  line L2590 (1.8106, 6.4539) -> (1.9776, 6.2732)
  line L2591 (1.9776, 6.2732) -> (1.8106, 6.0871)
  line L2592 (1.8106, 5.9825) -> (1.6436, 5.8018)
  line L2593 (1.6436, 5.8018) -> (1.8106, 5.6157)
  line L2594 (1.8106, 5.9825) -> (1.9776, 5.8018)
  line L2595 (1.9776, 5.8018) -> (1.8106, 5.6157)
  line L2596 (1.8106, 5.4909) -> (1.6436, 5.3102)
  line L2597 (1.6436, 5.3102) -> (1.8106, 5.124)
  line L2598 (1.8106, 5.4909) -> (1.9776, 5.3102)
  line L2599 (1.8106, 4.5539) -> (1.6436, 4.3732)
  line L2600 (1.8106, 4.5539) -> (1.9776, 4.3732)
  line L2601 (1.6436, 4.8325) -> (1.8106, 4.6463)
  line L2602 (1.9776, 4.8325) -> (1.8106, 4.6463)
  line L2603 (1.8106, 5.0132) -> (1.9776, 4.8325)
  line L2604 (1.9776, 5.3102) -> (1.8106, 5.124)
  line L2605 (1.8106, 5.0132) -> (1.6436, 4.8325)
  line L2606 (1.6436, 4.3732) -> (1.8106, 4.187)
  line L2607 (1.9776, 4.3732) -> (1.8106, 4.187)
  line L2608 (1.8106, 4.0906) -> (1.6436, 3.9099)
  line L2609 (1.8106, 4.0906) -> (1.9776, 3.9099)
  line L2610 (1.6436, 3.9099) -> (1.8106, 3.7237)
  line L2611 (1.9776, 3.9099) -> (1.8106, 3.7237)
  line L2612 (1.8106, 3.6252) -> (1.6436, 3.4445)
  line L2613 (1.8106, 3.6252) -> (1.9776, 3.4445)
  line L2614 (1.6436, 3.4445) -> (1.8106, 3.2584)
  line L2615 (1.9776, 3.4445) -> (1.8106, 3.2584)
  line L2616 (1.8106, 3.1357) -> (1.6436, 2.955)
  line L2617 (1.8106, 3.1357) -> (1.9776, 2.955)
  line L2618 (1.6436, 2.955) -> (1.8106, 2.7688)
  line L2619 (1.9776, 2.955) -> (1.8106, 2.7688)
  line L2620 (1.8106, 2.6703) -> (1.9776, 2.4896)
  line L2621 (1.8106, 2.6703) -> (1.6436, 2.4896)
  line L2622 (1.9776, 2.4896) -> (1.8106, 2.3035)
  line L2623 (1.6436, 2.4896) -> (1.8106, 2.3035)
  line L2624 (1.8106, 2.1808) -> (1.6436, 2.0001)
  line L2625 (1.8106, 2.1808) -> (1.9776, 2.0001)
  line L2626 (1.6436, 2.0001) -> (1.8106, 1.8139)
  line L2627 (1.9776, 2.0001) -> (1.8106, 1.8139)
  line L2628 (1.8106, 1.7094) -> (1.6436, 1.5287)
  line L2629 (1.8106, 1.7094) -> (1.9776, 1.5287)
  line L2630 (1.6436, 1.5287) -> (1.8106, 1.3425)
  line L2631 (1.9776, 1.5287) -> (1.8106, 1.3425)
  line L2632 (1.8106, 1.1085) -> (1.6436, 0.9278)
  line L2633 (1.6436, 0.9278) -> (1.8106, 0.7417)
  line L2634 (1.8106, 1.1085) -> (1.9776, 0.9278)
  line L2635 (1.6436, 0.4502) -> (1.8106, 0.264)
  line L2636 (1.9776, 0.4502) -> (1.8106, 0.264)
  line L2637 (1.8106, 0.6309) -> (1.9776, 0.4502)
  line L2638 (1.9776, 0.9278) -> (1.8106, 0.7417)
  line L2639 (1.8106, 0.6309) -> (1.6436, 0.4502)
  line L2640 (2.3274, 9.764) -> (2.1604, 9.5833)
  line L2641 (2.1604, 9.5833) -> (2.3274, 9.3971)
  line L2642 (2.3274, 9.764) -> (2.4944, 9.5833)
  line L2643 (2.3274, 8.827) -> (2.1604, 8.6463)
  line L2644 (2.3274, 8.827) -> (2.4944, 8.6463)
  line L2645 (2.4944, 9.1056) -> (2.3274, 8.9195)
  line L2646 (2.3274, 9.2863) -> (2.1604, 9.1056)
  line L2647 (2.3274, 9.2863) -> (2.4944, 9.1056)
  line L2648 (2.4944, 9.5833) -> (2.3274, 9.3971)
  line L2649 (2.1604, 9.1056) -> (2.3274, 8.9195)
  line L2650 (2.1604, 8.6463) -> (2.3274, 8.4602)
  line L2651 (2.4944, 8.6463) -> (2.3274, 8.4602)
  line L2652 (2.3274, 8.3637) -> (2.1604, 8.183)
  line L2653 (2.3274, 8.3637) -> (2.4944, 8.183)
  line L2654 (2.1604, 8.183) -> (2.3274, 7.9969)
  line L2655 (2.4944, 8.183) -> (2.3274, 7.9969)
  line L2656 (2.3274, 7.8983) -> (2.1604, 7.7177)
  line L2657 (2.1604, 7.7177) -> (2.3274, 7.5315)
  line L2658 (2.4944, 7.7177) -> (2.3274, 7.5315)
  line L2659 (2.3274, 7.8983) -> (2.4944, 7.7177)
  line L2660 (2.3274, 7.4088) -> (2.4944, 7.2281)
  line L2661 (2.3274, 7.4088) -> (2.1604, 7.2281)
  line L2662 (2.1604, 7.2281) -> (2.3274, 7.042)
  line L2663 (2.4944, 7.2281) -> (2.3274, 7.042)
  line L2664 (2.3274, 6.9434) -> (2.4944, 6.7628)
  line L2665 (2.4944, 6.7628) -> (2.3274, 6.5766)
  line L2666 (2.1604, 6.7628) -> (2.3274, 6.5766)
  line L2667 (2.3274, 6.9434) -> (2.1604, 6.7628)
  line L2668 (2.3274, 6.4539) -> (2.1604, 6.2732)
  line L2669 (2.3274, 6.4539) -> (2.4944, 6.2732)
  line L2670 (2.1604, 6.2732) -> (2.3274, 6.0871)
  line L2671 (2.4944, 6.2732) -> (2.3274, 6.0871)
  line L2672 (2.3274, 5.9825) -> (2.1604, 5.8018)
  line L2673 (2.3274, 5.9825) -> (2.4944, 5.8018)
  line L2674 (2.1604, 5.8018) -> (2.3274, 5.6157)
  line L2675 (2.4944, 5.8018) -> (2.3274, 5.6157)
  line L2676 (2.3274, 5.4909) -> (2.1604, 5.3102)
  line L2677 (2.3274, 5.4909) -> (2.4944, 5.3102)
  line L2678 (2.1604, 5.3102) -> (2.3274, 5.124)
  line L2679 (2.4944, 5.3102) -> (2.3274, 5.124)
  line L2680 (2.3274, 5.0132) -> (2.1604, 4.8325)
  line L2681 (2.3274, 5.0132) -> (2.4944, 4.8325)
  line L2682 (2.1604, 4.8325) -> (2.3274, 4.6463)
  line L2683 (2.4944, 4.8325) -> (2.3274, 4.6463)
  line L2684 (2.3274, 4.5539) -> (2.4944, 4.3732)
  line L2685 (2.3274, 4.5539) -> (2.1604, 4.3732)
  line L2686 (2.1604, 4.3732) -> (2.3274, 4.187)
  line L2687 (2.4944, 4.3732) -> (2.3274, 4.187)
  line L2688 (2.3274, 4.0906) -> (2.1604, 3.9099)
  line L2689 (2.3274, 4.0906) -> (2.4944, 3.9099)
  line L2690 (2.1604, 3.9099) -> (2.3274, 3.7237)
  line L2691 (2.4944, 3.9099) -> (2.3274, 3.7237)
  line L2692 (2.3274, 3.6252) -> (2.1604, 3.4445)
  line L2693 (2.3274, 3.6252) -> (2.4944, 3.4445)
  line L2694 (2.1604, 3.4445) -> (2.3274, 3.2584)
  line L2695 (2.4944, 3.4445) -> (2.3274, 3.2584)
  line L2696 (2.3274, 3.1357) -> (2.1604, 2.955)
  line L2697 (2.3274, 3.1357) -> (2.4944, 2.955)
  line L2698 (2.1604, 2.955) -> (2.3274, 2.7688)
  line L2699 (2.4944, 2.955) -> (2.3274, 2.7688)
  line L2700 (2.3274, 2.6703) -> (2.4944, 2.4896)
  line L2701 (2.3274, 2.6703) -> (2.1604, 2.4896)
  line L2702 (2.1604, 2.4896) -> (2.3274, 2.3035)
  line L2703 (2.4944, 2.4896) -> (2.3274, 2.3035)
  line L2704 (2.3274, 1.1085) -> (2.1604, 0.9278)
  line L2705 (2.3274, 1.1085) -> (2.4944, 0.9278)
  line L2706 (2.1604, 0.9278) -> (2.3274, 0.7417)
  line L2707 (2.3274, 0.6309) -> (2.4944, 0.4502)
  line L2708 (2.3274, 0.6309) -> (2.1604, 0.4502)
  line L2709 (2.1604, 0.4502) -> (2.3274, 0.264)
  line L2710 (2.4944, 0.4502) -> (2.3274, 0.264)
  line L2711 (2.4944, 0.9278) -> (2.3274, 0.7417)
  line L2712 (2.3274, 2.1808) -> (2.4944, 2.0001)
  line L2713 (2.3274, 2.1808) -> (2.1604, 2.0001)
  line L2714 (2.1604, 2.0001) -> (2.3274, 1.8139)
  line L2715 (2.4944, 2.0001) -> (2.3274, 1.8139)
  line L2716 (2.3274, 1.7094) -> (2.4944, 1.5287)
  line L2717 (2.3274, 1.7094) -> (2.1604, 1.5287)
  line L2718 (2.4944, 1.5287) -> (2.3274, 1.3425)
  line L2719 (2.1604, 1.5287) -> (2.3274, 1.3425)
  line L2720 (3.4111, 9.2863) -> (3.2441, 9.1056)
  line L2721 (3.4111, 9.2863) -> (3.5781, 9.1056)
  line L2722 (3.5781, 9.1056) -> (3.4111, 8.9195)
  line L2723 (3.2441, 9.1056) -> (3.4111, 8.9195)
  line L2724 (3.4111, 8.827) -> (3.5781, 8.6463)
  line L2725 (3.4111, 8.827) -> (3.2441, 8.6463)
  line L2726 (2.8943, 9.2863) -> (3.0613, 9.1056)
  line L2727 (2.8943, 9.2863) -> (2.7273, 9.1056)
  line L2728 (3.0613, 9.1056) -> (2.8943, 8.9195)
  line L2729 (2.7273, 9.1056) -> (2.8943, 8.9195)
  line L2730 (2.8943, 9.764) -> (2.7273, 9.5833)
  line L2731 (2.7273, 9.5833) -> (2.8943, 9.3971)
  line L2732 (3.0613, 9.5833) -> (2.8943, 9.3971)
  line L2733 (2.8943, 9.764) -> (3.0613, 9.5833)
  line L2734 (3.2441, 9.5833) -> (3.4111, 9.3971)
  line L2735 (3.5781, 9.5833) -> (3.4111, 9.3971)
  line L2736 (3.4111, 9.764) -> (3.2441, 9.5833)
  line L2737 (3.4111, 9.764) -> (3.5781, 9.5833)
  line L2738 (2.8943, 7.4088) -> (2.7273, 7.2281)
  line L2739 (2.7273, 7.2281) -> (2.8943, 7.042)
  line L2740 (2.8943, 6.4539) -> (3.0613, 6.2732)
  line L2741 (2.8943, 6.4539) -> (2.7273, 6.2732)
  line L2742 (3.0613, 6.2732) -> (2.8943, 6.0871)
  line L2743 (2.7273, 6.2732) -> (2.8943, 6.0871)
  line L2744 (3.4111, 5.9825) -> (3.5781, 5.8018)
  line L2745 (3.4111, 5.9825) -> (3.2441, 5.8018)
  line L2746 (3.5781, 5.8018) -> (3.4111, 5.6157)
  line L2747 (3.2441, 5.8018) -> (3.4111, 5.6157)
  line L2748 (2.8943, 5.9825) -> (3.0613, 5.8018)
  line L2749 (2.8943, 5.9825) -> (2.7273, 5.8018)
  line L2750 (3.0613, 5.8018) -> (2.8943, 5.6157)
  line L2751 (2.7273, 5.8018) -> (2.8943, 5.6157)
  line L2752 (3.2441, 4.8325) -> (3.4111, 4.6463)
  line L2753 (3.5781, 4.8325) -> (3.4111, 4.6463)
  line L2754 (2.8943, 5.0132) -> (3.0613, 4.8325)
  line L2755 (2.8943, 5.0132) -> (2.7273, 4.8325)
  line L2756 (3.4111, 4.5539) -> (3.5781, 4.3732)
  line L2757 (3.4111, 4.5539) -> (3.2441, 4.3732)
  line L2758 (3.0613, 4.8325) -> (2.8943, 4.6463)
  line L2759 (2.7273, 4.8325) -> (2.8943, 4.6463)
  line L2760 (2.8943, 4.5539) -> (3.0613, 4.3732)
  line L2761 (2.8943, 4.5539) -> (2.7273, 4.3732)
  line L2762 (3.0613, 3.4445) -> (2.8943, 3.2584)
  line L2763 (2.7273, 3.4445) -> (2.8943, 3.2584)
  line L2764 (2.8943, 3.6252) -> (3.0613, 3.4445)
  line L2765 (2.8943, 3.6252) -> (2.7273, 3.4445)
  line L2766 (2.7273, 3.9099) -> (2.8943, 3.7237)
  line L2767 (2.8943, 4.0906) -> (3.0613, 3.9099)
  line L2768 (2.8943, 4.0906) -> (2.7273, 3.9099)
  line L2769 (3.0613, 3.9099) -> (2.8943, 3.7237)
  line L2770 (2.8943, 8.827) -> (2.7273, 8.6463)
  line L2771 (2.7273, 8.6463) -> (2.8943, 8.4602)
  line L2772 (2.8943, 8.827) -> (3.0613, 8.6463)
  line L2773 (3.0613, 8.6463) -> (2.8943, 8.4602)
  line L2774 (2.8943, 8.3637) -> (2.7273, 8.183)
  line L2775 (2.7273, 8.183) -> (2.8943, 7.9969)
  line L2776 (2.8943, 8.3637) -> (3.0613, 8.183)
  line L2777 (3.5781, 8.6463) -> (3.4111, 8.4602)
  line L2778 (3.2441, 8.6463) -> (3.4111, 8.4602)
  line L2779 (3.4111, 8.3637) -> (3.5781, 8.183)
  line L2780 (3.5781, 8.183) -> (3.4111, 7.9969)
  line L2781 (3.2441, 8.183) -> (3.4111, 7.9969)
  line L2782 (3.0613, 8.183) -> (2.8943, 7.9969)
  line L2783 (3.4111, 8.3637) -> (3.2441, 8.183)
  line L2784 (2.8943, 7.8983) -> (2.7273, 7.7177)
  line L2785 (2.7273, 7.7177) -> (2.8943, 7.5315)
  line L2786 (2.8943, 7.4088) -> (3.0613, 7.2281)
  line L2787 (3.0613, 7.2281) -> (2.8943, 7.042)
  line L2788 (3.0613, 7.7177) -> (2.8943, 7.5315)
  line L2789 (2.8943, 7.8983) -> (3.0613, 7.7177)
  line L2790 (3.4111, 6.9434) -> (3.2441, 6.7628)
  line L2791 (3.4111, 6.9434) -> (3.5781, 6.7628)
  line L2792 (3.4111, 7.4088) -> (3.2441, 7.2281)
  line L2793 (3.5781, 7.2281) -> (3.4111, 7.042)
  line L2794 (3.2441, 7.7177) -> (3.4111, 7.5315)
  line L2795 (3.4111, 7.8983) -> (3.2441, 7.7177)
  line L2796 (3.4111, 7.8983) -> (3.5781, 7.7177)
  line L2797 (3.5781, 7.7177) -> (3.4111, 7.5315)
  line L2798 (3.4111, 7.4088) -> (3.5781, 7.2281)
  line L2799 (3.2441, 7.2281) -> (3.4111, 7.042)
  line L2800 (2.8943, 6.9434) -> (2.7273, 6.7628)
  line L2801 (2.7273, 6.7628) -> (2.8943, 6.5766)
  line L2802 (2.8943, 6.9434) -> (3.0613, 6.7628)
  line L2803 (3.0613, 6.7628) -> (2.8943, 6.5766)
  line L2804 (3.2441, 6.2732) -> (3.4111, 6.0871)
  line L2805 (3.5781, 6.2732) -> (3.4111, 6.0871)
  line L2806 (3.4111, 6.4539) -> (3.2441, 6.2732)
  line L2807 (3.4111, 6.4539) -> (3.5781, 6.2732)
  line L2808 (3.2441, 6.7628) -> (3.4111, 6.5766)
  line L2809 (3.5781, 6.7628) -> (3.4111, 6.5766)
  line L2810 (2.8943, 5.4909) -> (2.7273, 5.3102)
  line L2811 (2.7273, 5.3102) -> (2.8943, 5.124)
  line L2812 (2.8943, 5.4909) -> (3.0613, 5.3102)
  line L2813 (3.4111, 5.0132) -> (3.2441, 4.8325)
  line L2814 (3.0613, 5.3102) -> (2.8943, 5.124)
  line L2815 (3.2441, 5.3102) -> (3.4111, 5.124)
  line L2816 (3.5781, 5.3102) -> (3.4111, 5.124)
  line L2817 (3.4111, 5.4909) -> (3.2441, 5.3102)
  line L2818 (3.4111, 5.4909) -> (3.5781, 5.3102)
  line L2819 (3.4111, 5.0132) -> (3.5781, 4.8325)
  line L2820 (2.7273, 4.3732) -> (2.8943, 4.187)
  line L2821 (3.0613, 4.3732) -> (2.8943, 4.187)
  line L2822 (3.2441, 4.3732) -> (3.4111, 4.187)
  line L2823 (3.5781, 4.3732) -> (3.4111, 4.187)
  line L2824 (3.4111, 4.0906) -> (3.2441, 3.9099)
  line L2825 (3.4111, 4.0906) -> (3.5781, 3.9099)
  line L2826 (3.5781, 3.9099) -> (3.4111, 3.7237)
  line L2827 (3.4111, 3.6252) -> (3.2441, 3.4445)
  line L2828 (3.4111, 3.6252) -> (3.5781, 3.4445)
  line L2829 (3.2441, 3.4445) -> (3.4111, 3.2584)
  line L2830 (3.5781, 3.4445) -> (3.4111, 3.2584)
  line L2831 (3.2441, 3.9099) -> (3.4111, 3.7237)
  line L2832 (2.8943, 3.1357) -> (2.7273, 2.955)
  line L2833 (2.8943, 3.1357) -> (3.0613, 2.955)
  line L2834 (2.7273, 2.955) -> (2.8943, 2.7688)
  line L2835 (3.0613, 2.955) -> (2.8943, 2.7688)
  line L2836 (2.8943, 2.6703) -> (3.0613, 2.4896)
  line L2837 (2.8943, 2.6703) -> (2.7273, 2.4896)
  line L2838 (3.0613, 2.4896) -> (2.8943, 2.3035)
  line L2839 (2.7273, 2.4896) -> (2.8943, 2.3035)
  line L2840 (3.4111, 3.1357) -> (3.2441, 2.955)
  line L2841 (3.4111, 3.1357) -> (3.5781, 2.955)
  line L2842 (3.2441, 2.955) -> (3.4111, 2.7688)
  line L2843 (3.5781, 2.955) -> (3.4111, 2.7688)
  line L2844 (3.4111, 2.6703) -> (3.5781, 2.4896)
  line L2845 (3.4111, 2.6703) -> (3.2441, 2.4896)
  line L2846 (3.5781, 2.4896) -> (3.4111, 2.3035)
  line L2847 (3.2441, 2.4896) -> (3.4111, 2.3035)
  line L2848 (2.8943, 2.1808) -> (2.7273, 2.0001)
  line L2849 (2.8943, 2.1808) -> (3.0613, 2.0001)
  line L2850 (2.7273, 2.0001) -> (2.8943, 1.8139)
  line L2851 (3.0613, 2.0001) -> (2.8943, 1.8139)
  line L2852 (2.8943, 1.7094) -> (2.7273, 1.5287)
  line L2853 (2.8943, 1.7094) -> (3.0613, 1.5287)
  line L2854 (2.7273, 1.5287) -> (2.8943, 1.3425)
  line L2855 (3.0613, 1.5287) -> (2.8943, 1.3425)
  line L2856 (3.4111, 2.1808) -> (3.5781, 2.0001)
  line L2857 (3.4111, 2.1808) -> (3.2441, 2.0001)
  line L2858 (3.2441, 2.0001) -> (3.4111, 1.8139)
  line L2859 (3.5781, 2.0001) -> (3.4111, 1.8139)
  line L2860 (3.4111, 1.7094) -> (3.5781, 1.5287)
  line L2861 (3.4111, 1.7094) -> (3.2441, 1.5287)
  line L2862 (3.5781, 1.5287) -> (3.4111, 1.3425)
  line L2863 (3.2441, 1.5287) -> (3.4111, 1.3425)
  line L2864 (2.8943, 1.1085) -> (2.7273, 0.9278)
  line L2865 (2.7273, 0.9278) -> (2.8943, 0.7417)
  line L2866 (2.8943, 1.1085) -> (3.0613, 0.9278)
  line L2867 (2.7273, 0.4502) -> (2.8943, 0.264)
  line L2868 (3.0613, 0.4502) -> (2.8943, 0.264)
  line L2869 (2.8943, 0.6309) -> (3.0613, 0.4502)
  line L2870 (3.0613, 0.9278) -> (2.8943, 0.7417)
  line L2871 (2.8943, 0.6309) -> (2.7273, 0.4502)
  line L2872 (3.4111, 1.1085) -> (3.2441, 0.9278)
  line L2873 (3.4111, 1.1085) -> (3.5781, 0.9278)
  line L2874 (3.2441, 0.9278) -> (3.4111, 0.7417)
  line L2875 (3.5781, 0.9278) -> (3.4111, 0.7417)
  line L2876 (3.4111, 0.6309) -> (3.5781, 0.4502)
  line L2877 (3.4111, 0.6309) -> (3.2441, 0.4502)
  line L2878 (3.2441, 0.4502) -> (3.4111, 0.264)
  line L2879 (3.5781, 0.4502) -> (3.4111, 0.264)
  point P0 (14, 10)
  constraints: 5760 end point